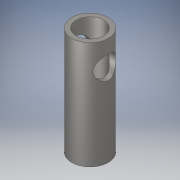
# Autodesk Inventor part: Piston
Saved by Autodesk Inventor 2018 (Build 220112000, 112)
## iProperties
Created: 2017-09-20
Part Number: Piston
Material: Generic
Document SubType Name: Modeling
Designer: Intel
Density: 1 g/cm^3
Appearance: Stainless - Brushed
Author: Intel
Autodesk Inventor part; units mm, degrees
note: some values were not read from the file. Chosen so that the rebuilt part matches the saved one: second side of "Extrusion1".
ref_plane "YZ Plane" through (0, 0, 0) normal (1, 0, 0) x (0, 1, 0)
ref_plane "XZ Plane" through (0, 0, 0) normal (0, 1, 0) x (-1, 0, 0)
ref_plane "XY Plane" through (0, 0, 0) normal (0, 0, 1) x (1, 0, 0)
sketch "Sketch1" plane through (0, 0, 0) normal (0, 1, 0) x (-1, 0, 0)
  circle A0 centre (0, 0) radius 6.35
  dimension "d0" = 12.7
  constraints: 1 centre point, 1 coincident
  measures "d0" diameter of A0
extrude "Extrusion1" add sketch "Sketch1" along normal blind 37.4904
sketch "Sketch3" plane through (0, 37.4904, 0) normal (0, 1, 0) x (1, 0, 0)
  circle A0 centre (0, 0) radius 4.7625
  dimension "d10" = 9.525
  constraints: 1 centre point, 1 coincident
  measures "d10" diameter of A0
extrude "Extrusion3" cut sketch "Sketch3" against normal blind 31.75
sketch "Sketch4" plane through (0, 0, 0) normal (1, 0, 0) x (0, 1, 0)
  line L0 (37.4904, -6.35) -> (37.4904, 6.35) projected
  line L1 (0, -6.35) -> (37.4904, -6.35) projected
  line L2 (0, 6.35) -> (37.4904, 6.35) projected
  line L3 (0, 6.35) -> (0, -6.35) projected
  circle A0 centre (28.7782, 0) radius 3.9624
  point P0 (0, 0)
  dimension "d13" = 7.9248
  dimension "d14" = 28.7782
  dimension "d15" = 6.35
  constraints: 1 centre point
  measures "d13" diameter of A0
  measures "d14" distance from line of L3 A0.centre
  measures "d15" distance from line of L1 A0.centre
extrude "Extrusion4" cut sketch "Sketch4" along normal mid plane 25.4 contours A0
body "Solid1"
